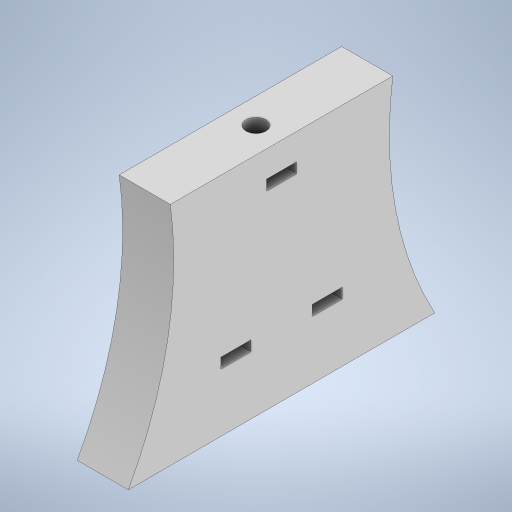
# Autodesk Inventor part: cuerpo_obj1
Saved by Autodesk Inventor 2023.2 (Build 272271030, 271C)
## iProperties
Created: 2023-02-25
Part Number: cuerpo_obj1
Material: Generic
Document SubType Name: Modeling
Designer: Cris Pat
Density: 1 g/cm^3
Appearance: Default
Author: Cris Pat
Autodesk Inventor part; units mm, degrees
ref_plane "YZ Plane" through (0, 0, 0) normal (1, 0, 0) x (0, 1, 0)
ref_plane "XZ Plane" through (0, 0, 0) normal (0, 1, 0) x (-1, 0, 0)
ref_plane "XY Plane" through (0, 0, 0) normal (0, 0, 1) x (1, 0, 0)
sketch "Sketch1" plane through (0, 0, 0) normal (1, 0, 0) x (0, 1, 0)
  arc A0 (31, -30.4818) -> (-31, -42) centre (17.3336, -129.5435) ccw
  line L0 (-31, 42) -> (31, 42) construction
  line L1 (31, 42) -> (31, -42) construction
  line L2 (31, -42) -> (-31, -42) construction
  line L3 (-31, -42) -> (-31, 42)
  line L4 (31, 0) -> (-31, 0) construction
  arc A1 (-31, 42) -> (31, 30.4818) centre (17.3336, 129.5435) ccw
  line L5 (31, 30.4818) -> (31, -30.4818)
  point P0 (0, 0)
  point P1 (0, 42)
  dimension "d0" = 200
  dimension "d1" = 62
  dimension "d2" = 84
  dimension "d3" = 60.9635
  constraints: 12 end point, 5 point on circle, 3 midpoint, 2 centre point, 2 parallel, 2 point on line, 1 collinear, 1 horizontal, 1 horizontal alignment, 1 perpendicular, 1 symmetric about line, 1 vertical alignment, 1 other
  measures "d0" diameter of A0
  measures "d1" distance of L1.end L2.end
  measures "d2" distance of L0.end L1.end
  measures "d3" distance of A1.end L5.end
extrude "Extrusion1" add sketch "Sketch1" along normal mid plane 14
sketch "Sketch2" plane through (7, 0, 0) normal (1, 0, 0) x (0, 0, -1)
  arc A0 (-42, -31) -> (-30.4818, 31) centre (-129.5435, 17.3336) ccw construction
  line L0 (-42, -31) -> (42, -31) construction
  arc A1 (30.4818, 31) -> (42, -31) centre (129.5435, 17.3336) ccw construction
  line L1 (30.4818, 31) -> (-30.4818, 31) construction
  line L2 (-16.6, -12.2) -> (-8.4, -12.2)
  line L3 (-8.4, -12.2) -> (-8.4, -15)
  line L4 (-8.4, -15) -> (-16.6, -15)
  line L5 (-16.6, -15) -> (-16.6, -12.2)
  line L6 (0, 0) -> (0, -31) construction
  line L7 (-42, -31) -> (42, -31) construction
  line L8 (16.6, -12.2) -> (8.4, -12.2)
  line L9 (8.4, -12.2) -> (8.4, -15)
  line L10 (8.4, -15) -> (16.6, -15)
  line L11 (16.6, -15) -> (16.6, -12.2)
  line L12 (-4.1, 23.8) -> (4.1, 23.8)
  line L13 (4.1, 23.8) -> (4.1, 21)
  line L14 (4.1, 21) -> (-4.1, 21)
  line L15 (-4.1, 21) -> (-4.1, 23.8)
  point P0 (12.5, -12.2)
  point P1 (-12.5, -12.2)
  point P2 (0, 23.8)
  dimension "d6" = 8.2
  dimension "d7" = 2.8
  dimension "d8" = 16
  dimension "d9" = 25
  dimension "d16" = 8.2
  dimension "d17" = 2.8
  dimension "d19" = 10
  constraints: 26 end point, 4 midpoint, 4 parallel, 4 symmetric about line, 2 horizontal, 2 perpendicular, 1 vertical alignment
  measures "d6" distance of L3.end L4.end
  measures "d7" distance of L2.end L3.end
  measures "d8" distance between parallel lines of L0 L4
  measures "d9" distance of point (12.5, -12.2) point (-12.5, -12.2)
  measures "d16" distance of L13.end L14.end
  measures "d17" distance of L12.end L13.end
  measures "d19" distance between parallel lines of L14 L1
extrude "Extrusion2" cut sketch "Sketch2" against normal through all
sketch "Sketch3" plane through (-7, -31, -42) normal (0, -1, 0) x (1, 0, 0)
  line L0 (0, 0) -> (14, 0) construction
  line L1 (14, 84) -> (14, 0) construction
  line L2 (0, 84) -> (14, 84) construction
  line L3 (0, 0) -> (0, 84) construction
  line L4 (14, 42) -> (0, 42) construction
  line L5 (0, 0) -> (0, 84) construction
  line L6 (0, 84) -> (14, 84) construction
  line L7 (7, 84) -> (7, 0) construction
  line L8 (0, 0) -> (14, 0) construction
  circle A0 centre (7, 54.5) radius 2.75
  circle A1 centre (7, 29.5) radius 2.75
  point P0 (7, 42)
  dimension "d12" = 5.5
  dimension "d13" = 25
  constraints: 4 end point, 4 midpoint, 2 centre point, 1 point on line, 1 symmetric about line, 1 other
  measures "d12" diameter of A0
  measures "d13" distance of A1.centre A0.centre
extrude "Extrusion3" cut sketch "Sketch3" against normal blind 25
sketch "Sketch4" plane through (-7, 31, 30.4818) normal (0, 1, 0) x (1, 0, 0)
  line L0 (14, 0) -> (0, 0) construction
  line L1 (14, 60.9635) -> (14, 0) construction
  line L2 (0, 60.9635) -> (14, 60.9635) construction
  line L3 (0, 0) -> (0, 60.9635) construction
  line L4 (0, 30.4818) -> (14, 30.4818) construction
  line L5 (14, 26.3818) -> (14, 34.5818) construction
  line L6 (14, 0) -> (0, 0) construction
  line L7 (7, 0) -> (7, 60.9635) construction
  line L8 (0, 60.9635) -> (14, 60.9635) construction
  circle A0 centre (7, 30.4818) radius 2.75
  dimension "d20" = 5.5
  constraints: 4 end point, 4 midpoint, 1 centre point, 1 coincident
  measures "d20" diameter of A0
extrude "Extrusion4" cut sketch "Sketch4" against normal blind 15
body "Solid1"
